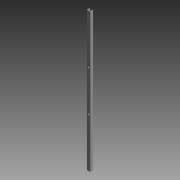
# Autodesk Inventor part: stab
Saved by Autodesk Inventor 2013 (Build 170138000, 138)
## iProperties
Created: 2012-10-24
Part Number: stab
Material: Allgemein
Document SubType Name: Modeling
Designer: fivef
Density: 1 g/cm^3
Author: fivef
Autodesk Inventor part; units mm, degrees
ref_plane "YZ Plane" through (0, 0, 0) normal (1, 0, 0) x (0, 1, 0)
ref_plane "XZ Plane" through (0, 0, 0) normal (0, 1, 0) x (-1, 0, 0)
ref_plane "XY Plane" through (0, 0, 0) normal (0, 0, 1) x (1, 0, 0)
sketch "Skizze1" plane through (0, 0, 0) normal (0, 0, 1) x (1, 0, 0)
  line L0 (0, 0) -> (4.6893, 0)
  line L1 (4.6893, 0) -> (4.6893, 8.2)
  line L2 (4.6893, 8.2) -> (3.3893, 8.2)
  line L3 (3.3893, 8.2) -> (3.3893, 1.3)
  line L4 (3.3893, 1.3) -> (-4.1107, 1.3)
  line L5 (-4.1107, 1.3) -> (-4.1107, 8.2)
  line L6 (-4.1107, 8.2) -> (-5.4107, 8.2)
  line L7 (-5.4107, 8.2) -> (-5.4107, 0)
  line L8 (-5.4107, 0) -> (0, 0)
  line L9 (0, 8.5935) -> (0, -2.965) construction
  dimension "d0" = 10.1
  dimension "d2" = 8.2
  dimension "d3" = 8.2
  dimension "d4" = 1.3
  dimension "d5" = 1.3
  dimension "d6" = 1.3
  constraints: 20 end point, 6 parallel, 1 point on line, 1 vertical
  measures "d0" distance between parallel lines of L1 L7
  measures "d2" distance of L0.end L1.end
  measures "d3" distance of L6.end L7.end
  measures "d4" distance of L5.end L6.end
  measures "d5" distance between parallel lines of L8 L4
  measures "d6" distance of L1.end L2.end
extrude "Extrusion1" add sketch "Skizze1" along normal mid plane 410
sketch "Skizze2" plane through (-5.4107, 0, 205) normal (0, -1, 0) x (1, 0, 0)
  point P0 (5.4107, -205)
  point P1 (5.4107, -145)
  point P2 (5.4107, -265)
  dimension "d9" = 60
  dimension "d10" = 60
  dimension "d11" = 0
  dimension "d12" = 0
  measures "d9" distance of point (5.411, -145) point (5.411, -205)
  measures "d10" distance of point (5.411, -205) point (5.411, -265)
  measures "d11" horizontal distance of point (5.411, -145) point (5.411, -205)
  measures "d12" horizontal distance of point (5.411, -205) point (5.411, -265)
hole "Bohrung1" at (0, 0, 60) at (0, 0, -60) direction (0, 1, 0) diameter 4.3 end through all
